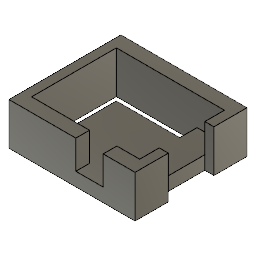
case (Autodesk Fusion 360 design; units mm, degrees)
Autodesk Fusion 360 part; units mm, degrees
sketch "Sketch1" plane through (0, 0, 0) normal (0, 0, 1) x (1, 0, 0) in component "case"
  line L0 (0, 0) -> (23.7, 0)
  line L1 (23.7, 0) -> (23.7, 18.6)
  line L2 (23.7, 18.6) -> (0, 18.6)
  line L3 (0, 18.6) -> (0, 0)
  circle A0 centre (21, 16.05) radius 1.5
  circle A1 centre (21, 2.55) radius 1.5
  line L4 (21, 16.05) -> (21, 2.55) construction
  line L5 (23.7, 9.3) -> (0, 9.3) construction
  line L6 (3.75, 0) -> (3.75, 14.85)
  line L7 (3.75, 14.85) -> (17.7, 14.85)
  line L8 (17.7, 14.85) -> (17.7, 18.6)
  line L9 (-2, 21.6) -> (25.7, 21.6)
  line L10 (25.7, 21.6) -> (25.7, -3)
  line L11 (25.7, -3) -> (-2, -3)
  line L12 (-2, -3) -> (-2, 21.6)
  line L13 (11.85, -3) -> (11.85, 21.6) construction
  line L14 (18.7, 0) -> (18.7, -3)
  line L15 (12.7, 0) -> (12.7, -3)
  line L16 (23.7, 14.3) -> (25.7, 14.3)
  line L17 (23.7, 4.3) -> (25.7, 4.3)
  line L18 (24.7, 14.3) -> (24.7, 4.3) construction
  point P0 (21, 9.3)
  point P1 (24.7, 9.3)
  dimension "d1" = 23.7
  dimension "d2" = 18.6
  dimension "d3" = 3
  dimension "d4" = 3
  dimension "d5" = 16.5
  dimension "d6" = 1.2
  dimension "d7" = 6
  dimension "d8" = 3.75
  dimension "d12" = 3
  dimension "d13" = 2
  dimension "d14" = 5
  dimension "d15" = 6
  dimension "d18" = 10
  dimension "d19" = 3.75
  constraint horizontal L0
  constraint vertical L1
  constraint horizontal L2
  constraint vertical L3
  constraint coincident L0.start L3.end
  constraint coincident A0.centre L4.start
  constraint coincident A1.centre L4.end
  constraint parallel L1 L4
  constraint midpoint L1 L5.start
  constraint midpoint L3 L5.end
  constraint midpoint L4 P0
  constraint coincident L5 P0
  constraint perpendicular L2 L6
  constraint perpendicular L6 L7
  constraint perpendicular L0 L8
  constraint horizontal L9
  constraint vertical L10
  constraint horizontal L11
  constraint vertical L12
  constraint midpoint L11 L13.start
  constraint midpoint L9 L13.end
  constraint midpoint L5 L13
  constraint coincident L0 L14.start
  constraint coincident L11 L14.end
  constraint perpendicular L11 L14
  constraint coincident L0 L15.start
  constraint coincident L11 L15.end
  constraint perpendicular L11 L15
  constraint coincident L1 L16.start
  constraint coincident L10 L16.end
  constraint perpendicular L1 L16
  constraint coincident L1 L17.start
  constraint coincident L10 L17.end
  constraint perpendicular L10 L17
  constraint midpoint L16 L18.start
  constraint midpoint L17 L18.end
  constraint midpoint L18 P1
  constraint coincident L5 P1
  constraint coincident L2 L8.end
  constraint coincident L0 L6.start
  measures "d1" distance of L0.start L0.end
  measures "d2" distance of L0.start L2.end
  measures "d3" diameter of A0
  measures "d4" diameter of A1
  measures "d6" distance of L1 A1
  measures "d7" distance of L1 L8
  measures "d8" distance of L3 L6
  measures "d12" distance of L2 L9
  measures "d13" distance of L1 L10
  measures "d14" distance of L1 L14
  measures "d15" distance of L14 L15
  measures "d18" distance of L16 L17
  measures "d19" distance of L7.end L8.end
extrude "Extrude1" add sketch "Sketch1" against normal blind 3 contours L0 L1 L2 L3 L9 L10 L11 L12 L15 L16 | L0 L1 L2 L6 L7 L8 | L0 L11 L14 L15 | L0 L1 L10 L11 L14 L17 | A0 | A1 in component "case"
extrude "Extrude2" add sketch "Sketch1" along normal blind 6.3 contours L0 L1 L2 L3 L9 L10 L11 L12 L15 L16 | L0 L1 L10 L11 L14 L17 in component "case"
component "case" placed x (1, 0, 0) y (0, 1, 0) z (0, 0, 1) at (0, 0, 0)
equation "d19 = d8"
